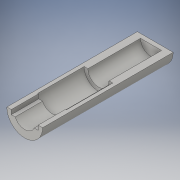
# Autodesk Inventor part: Snap-Twist Idea F
Saved by Autodesk Inventor 2016 (Build 200138000, 138)
## iProperties
Created: 2015-08-07
Part Number: Snap-Twist Idea F
Material: Generic
Document SubType Name: Modeling
Designer: Nancy
Density: 1 g/cm^3
Appearance: Default
Mass: 0.0663045 g
Surface Area: 2.18833 cm^2
Volume: 0.0663045 cm^3
Author: Nancy
Autodesk Inventor part; units mm, degrees
ref_plane "YZ Plane" through (0, 0, 0) normal (1, 0, 0) x (0, 1, 0)
ref_plane "XZ Plane" through (0, 0, 0) normal (0, 1, 0) x (-1, 0, 0)
sketch "Sketch1" plane through (0, 0, 0) normal (0, 0, 1) x (1, 0, 0)
  circle A0 centre (0, 0) radius 2.159
  dimension "d0" = 4.318
  constraints: 1 centre point, 1 coincident
  measures "d0" diameter of A0
extrude "Extrusion1" add sketch "Sketch1" along normal blind 15.748
sketch "Sketch2" plane through (0, 0, 15.748) normal (0, 0, 1) x (1, 0, 0)
  circle A0 centre (0, 0) radius 1.275
  dimension "d23" = 2.55
  constraints: 1 centre point
  measures "d23" diameter of A0
extrude "Extrusion2" cut sketch "Sketch2" against normal blind 15.24
sketch "Sketch6" plane through (0, 0, 15.748) normal (0, 0, 1) x (1, 0, 0)
  line L0 (-1.6256, 0.5334) -> (1.6256, 0.5334)
  line L1 (1.6256, 0.5334) -> (1.6256, -0.5334)
  line L2 (1.6256, -0.5334) -> (-1.6256, -0.5334)
  line L3 (-1.6256, -0.5334) -> (-1.6256, 0.5334)
  point P0 (0, 0)
  dimension "d24" = 0.5334
  dimension "d25" = 0.5334
  dimension "d26" = 1.6256
  dimension "d27" = 1.6256
  constraints: 8 end point, 2 parallel, 1 horizontal, 1 perpendicular
  measures "d24" distance from line of point (0, 0) L0
  measures "d25" distance from line of point (0, 0) L2
  measures "d26" distance from line of point (0, 0) L1
  measures "d27" distance from line of point (0, 0) L3
extrude "Extrusion6" cut sketch "Sketch6" against normal blind 8.89
ref_plane "Work Plane2" through (0, 0, 6.858) normal (0, 0, 1) x (1, 0, 0)
sketch "Sketch7" plane through (0, 0, 6.858) normal (0, 0, 1) x (1, 0, 0)
  line L0 (1.6428, -0.5334) -> (1.1581, -0.5334)
  line L1 (-1.6428, 0.5334) -> (-0.5334, 0.5334)
  arc A0 (1.6428, -0.5334) -> (-0.5334, 1.6428) centre (0, 0) ccw
  arc A1 (-1.6428, 0.5334) -> (0.5334, -1.6428) centre (0, 0) ccw
  line L2 (1.6256, -0.5334) -> (0.5334, -0.5334)
  line L3 (0.5334, -0.5334) -> (0.5334, -1.6428)
  line L4 (-0.5334, 0.5334) -> (-0.5334, 1.6428)
  constraints: 10 end point, 4 point on circle, 2 centre point, 2 parallel, 1 coincident, 1 horizontal, 1 point on line
extrude "Extrusion7" cut sketch "Sketch7" along normal blind 5.588
sketch "Sketch8" plane through (0, 0, 0) normal (0, 0, -1) x (-1, 0, 0)
  line L0 (-3.8846, 4.0845) -> (4.056, 4.0845)
  line L1 (4.056, 4.0845) -> (4.056, 0)
  line L2 (4.056, 0) -> (-3.8846, 0)
  line L3 (-3.8846, 0) -> (-3.8846, 4.0845)
  point P0 (0, 0)
  constraints: 8 end point, 2 parallel, 1 horizontal, 1 perpendicular
extrude "Extrusion8" cut sketch "Sketch8" against normal blind 25.4
body "Solid1"
